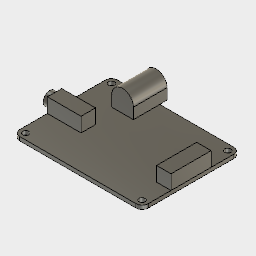
1752 MAX9744 (Autodesk Fusion 360 design; units mm, degrees)
Autodesk Fusion 360 part; units mm, degrees
sketch "Sketch1" plane through (0, 0, 0) normal (0, 0, 1) x (1, 0, 0)
  line L0 (0, 0) -> (53.34, 0)
  line L1 (53.34, 0) -> (53.34, 40.64)
  line L2 (53.34, 40.64) -> (0, 40.64)
  line L3 (0, 40.64) -> (0, 0)
  circle A0 centre (2.54, 2.54) radius 1.25
  line L4 (26.67, 40.64) -> (26.67, 0) construction
  line L5 (53.34, 20.32) -> (0, 20.32) construction
  circle A1 centre (50.8, 2.54) radius 1.25
  circle A2 centre (2.54, 38.1) radius 1.25
  circle A3 centre (50.8, 38.1) radius 1.25
  line L6 (0, 20.02) -> (14, 20.02)
  line L7 (14, 20.02) -> (14, 14.02)
  line L8 (14, 14.02) -> (0, 14.02)
  line L9 (0, 14.02) -> (0, 20.02)
  line L10 (14, 17.02) -> (0, 17.02) construction
  line L11 (11.09, 43.64) -> (20.09, 43.64)
  line L12 (20.09, 43.64) -> (20.09, 29.64)
  line L13 (20.09, 29.64) -> (11.09, 29.64)
  line L14 (11.09, 29.64) -> (11.09, 43.64)
  line L15 (15.59, 43.64) -> (15.59, 29.64) construction
  line L16 (53.34, 12) -> (47.34, 12)
  line L17 (47.34, 12) -> (47.34, 28.64)
  line L18 (47.34, 28.64) -> (53.34, 28.64)
  line L19 (53.34, 28.64) -> (53.34, 12)
  line L20 (53.34, 12) -> (47.34, 28.64) construction
  line L21 (47.34, 12) -> (53.34, 28.64) construction
  point P0 (50.34, 20.32)
  dimension "d1" = 53.34
  dimension "d2" = 40.64
  dimension "d3" = 2.5
  dimension "d4" = 2.54
  dimension "d5" = 2.54
  dimension "d9" = 14
  dimension "d10" = 6
  dimension "d11" = 17.02
  dimension "d12" = 9
  dimension "d13" = 14
  dimension "d14" = 15.59
  dimension "d15" = 3
  dimension "d24" = 16.64
  dimension "d25" = 6
  measures "d1" distance of L0.start L0.end
  measures "d2" distance of L0.start L2.end
  measures "d3" diameter of A0
  measures "d4" distance of L3 A0.centre
  measures "d5" distance of L0 A0.centre
  measures "d9" distance of L6.start L6.end
  measures "d10" distance of L6.start L8.end
  measures "d11" distance of L0 L10
  measures "d12" distance of L11.start L11.end
  measures "d13" distance of L11.start L13.end
  measures "d14" distance of L3 L15
  measures "d15" distance of L2 L11
  measures "d24" distance of L16.end L17.end
  measures "d25" distance of L17.end L18.end
extrude "Extrude1" add sketch "Sketch1" against normal blind 1.6 contours L0 L1 L2 L3 L6 L7 L8 L12 L13 L14 L16 L17 L18 | L3 L6 L7 L8 L9 | L1 L16 L17 L18 L19 | L2 L12 L13 L14 makes body 1
fillet "Fillet1" radius 2.54 4 edges at (53.34, 0, -0.8) (53.34, 40.64, -0.8) (0, 40.64, -0.8) (0, 0, -0.8) on bodies 1
extrude "Extrude2" add sketch "Sketch1" along normal blind 6 separate body contours L3 L6 L7 L8 L9 makes body 2
sketch "Sketch2" plane through (0, 0, 0) normal (-1, 0, 0) x (0, -1, 0)
  line L0 (-20.02, 0) -> (-14.02, 0)
  line L1 (-14.02, 0) -> (-14.02, 6)
  line L2 (-14.02, 6) -> (-20.02, 6)
  line L3 (-20.02, 6) -> (-20.02, 0)
  line L4 (-17.02, 6) -> (-17.02, 0) construction
  line L5 (-20.02, 3) -> (-14.02, 3) construction
  circle A0 centre (-17.02, 3) radius 2.75
  point P0 (-17.02, 0)
  dimension "d18" = 5.5
  measures "d18" diameter of A0
extrude "Extrude3" add sketch "Sketch2" along normal blind 2 contours A0 bodies 2
extrude "Extrude4" add sketch "Sketch1" along normal blind 9 separate body contours L2 L11 L12 L14 | L2 L12 L13 L14 makes body 3
fillet "Fillet2" radius 4.5 2 edges at (11.09, 36.64, 9) (20.09, 36.64, 9) on bodies 3
extrude "Extrude5" add sketch "Sketch1" along normal blind 6 separate body contours L1 L16 L17 L18 L19 makes body 4
